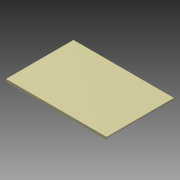
# Autodesk Inventor part: SidePanelNarrow
Saved by Autodesk Inventor 2015 (Build 190159000, 159)
## iProperties
Created: 2015-04-21
Part Number: SidePanelNarrow
Material: Nylon 6
Document SubType Name: Modeling
Designer: Akovo_000
Mass: 17.0375 g
Surface Area: 300.154 cm^2
Volume: 15.2121 cm^3
Density: 1.12 g/cm^3
Appearance: Nylon 6
Author: Akovo_000
Autodesk Inventor part; units mm, degrees
ref_plane "YZ Plane" through (0, 0, 0) normal (1, 0, 0) x (0, 1, 0)
ref_plane "XZ Plane" through (0, 0, 0) normal (0, 1, 0) x (-1, 0, 0)
ref_plane "XY Plane" through (0, 0, 0) normal (0, 0, 1) x (1, 0, 0)
sketch "PanelBody" plane through (0, 0, 0) normal (0, 0, 1) x (1, 0, 0)
  line L0 (-106.0995, -38.4223) -> (33.9005, -38.4223)
  line L1 (33.9005, -38.4223) -> (33.9005, -132.4223)
  line L2 (33.9005, -132.4223) -> (-106.0995, -132.4223)
  line L3 (-106.0995, -132.4223) -> (-106.0995, -38.4223)
  dimension "d1" = 140
  dimension "d2" = 94
  constraints: 8 end point, 2 parallel, 1 horizontal, 1 perpendicular
  measures "d1" distance of L1.end L2.end
  measures "d2" distance of L0.end L1.end
extrude "PanelFace" add sketch "PanelBody" along normal blind 2
sketch "SideHooks" plane through (-106.0995, -132.4223, 0) normal (-1, 0, 0) x (0, 0, 1)
  line L0 (0, 94) -> (-1.9, 94)
  line L1 (-1.9, 94) -> (-1.9, 92.1)
  line L2 (-1.9, 92.1) -> (0, 92.1)
  line L3 (0, 92.1) -> (0, 94)
  line L4 (0, 0) -> (-1.9, 0)
  line L5 (-1.9, 0) -> (-1.9, 1.9)
  line L6 (-1.9, 1.9) -> (0, 1.9)
  line L7 (0, 1.9) -> (0, 0)
  point P0 (0, 132.4223)
  dimension "d33" = 1.9
  constraints: 16 end point, 4 parallel, 3 equal length, 2 horizontal, 2 perpendicular
  measures "d33" distance of L5.end L6.end
extrude "Corners" add sketch "SideHooks" against normal blind 140
sketch "Sketch3" plane through (33.9005, -38.4223, -1.9) normal (0, 0, -1) x (-1, 0, 0)
  line L0 (0, -94) -> (140, -94) construction
  line L1 (140, -94) -> (140, 0) construction
  line L2 (140, 0) -> (0, 0) construction
  line L3 (0, 0) -> (0, -94) construction
  line L4 (137.5, -91.5) -> (133.8633, -91.5) construction
  line L5 (72.5, -86.5) -> (72.5, -56.6362)
  line L6 (137.5, -54.5) -> (137.5, -85.1873)
  line L7 (137.5, -2.5) -> (133.8633, -2.5) construction
  line L8 (72.5, -7.5) -> (72.5, -37.3638)
  line L9 (137.5, -39.5) -> (137.5, -8.8127)
  line L10 (2.5, -2.5) -> (6.1367, -2.5) construction
  line L11 (67.5, -7.5) -> (67.5, -37.3638)
  line L12 (2.5, -39.5) -> (2.5, -8.8127)
  line L13 (2.5, -91.5) -> (6.1367, -91.5) construction
  line L14 (67.5, -86.5) -> (67.5, -56.6362)
  line L15 (2.5, -54.5) -> (2.5, -85.1873)
  line L16 (72.5, -2.5) -> (67.5, -2.5) construction
  line L17 (2.5, -44.5) -> (2.5, -49.5) construction
  line L18 (67.5, -91.5) -> (72.5, -91.5) construction
  line L19 (137.5, -44.5) -> (137.5, -49.5) construction
  line L20 (135.2172, -7.5332) -> (79.3341, -41.7204)
  line L21 (74.7828, -38.6434) -> (129.3198, -5.2796)
  line L22 (65.2172, -38.6434) -> (10.6802, -5.2796)
  line L23 (60.6659, -41.7204) -> (4.7828, -7.5332)
  line L24 (11.4629, -2.5) -> (62.5, -2.5)
  line L25 (2.5, -6.1367) -> (2.5, -2.5) construction
  line L26 (80.1169, -44.5) -> (132.5, -44.5)
  line L27 (137.5, -6.1367) -> (137.5, -2.5) construction
  line L28 (128.5371, -2.5) -> (77.5, -2.5)
  line L29 (59.8831, -44.5) -> (7.5, -44.5)
  line L30 (135.2172, -86.4668) -> (79.3341, -52.2796)
  line L31 (74.7828, -55.3566) -> (129.3198, -88.7204)
  line L32 (65.2172, -55.3566) -> (10.6802, -88.7204)
  line L33 (4.7828, -86.4668) -> (60.6659, -52.2796)
  line L34 (80.1169, -49.5) -> (132.5, -49.5)
  line L35 (59.8831, -49.5) -> (7.5, -49.5)
  line L36 (2.5, -87.8633) -> (2.5, -91.5) construction
  line L37 (11.4629, -91.5) -> (62.5, -91.5)
  line L38 (128.5371, -91.5) -> (77.5, -91.5)
  line L39 (137.5, -87.8633) -> (137.5, -91.5) construction
  line L40 (140, -94) -> (0, -94) projected
  line L41 (140, 0) -> (0, 0) projected
  line L42 (0, -1.9) -> (0, -92.1) projected
  line L43 (140, 0) -> (140, -1.9) projected
  line L44 (103.0028, -27.2408) -> (100.3935, -22.9756) construction
  line L45 (91.7427, -59.8707) -> (89.1334, -64.1358) construction
  line L46 (57.5593, -60.0415) -> (54.95, -55.7763) construction
  line L47 (48.3721, -34.1995) -> (50.9813, -29.9344) construction
  line L48 (74.7906, -49.5) -> (65.2094, -49.5) construction
  line L49 (65.2094, -44.5) -> (74.7906, -44.5) construction
  line L50 (72.5, -53.9601) -> (72.5, -40.0399) construction
  line L51 (67.5, -53.9601) -> (67.5, -40.0399) construction
  arc A0 (77.5, -2.5) -> (72.5, -7.5) centre (77.5, -7.5) ccw
  arc A1 (67.5, -7.5) -> (62.5, -2.5) centre (62.5, -7.5) ccw
  arc A2 (72.5, -86.5) -> (77.5, -91.5) centre (77.5, -86.5) ccw
  arc A3 (62.5, -91.5) -> (67.5, -86.5) centre (62.5, -86.5) ccw
  arc A4 (2.5, -39.5) -> (7.5, -44.5) centre (7.5, -39.5) ccw
  arc A5 (7.5, -49.5) -> (2.5, -54.5) centre (7.5, -54.5) ccw
  arc A6 (137.5, -54.5) -> (132.5, -49.5) centre (132.5, -54.5) ccw
  arc A7 (132.5, -44.5) -> (137.5, -39.5) centre (132.5, -39.5) ccw
  arc A8 (80.1169, -49.5) -> (79.3341, -52.2796) centre (80.1169, -51) ccw
  arc A9 (74.7828, -55.3566) -> (72.5, -56.6362) centre (74, -56.6362) ccw
  arc A10 (67.5, -56.6362) -> (65.2172, -55.3566) centre (66, -56.6362) ccw
  arc A11 (60.6659, -52.2796) -> (59.8831, -49.5) centre (59.8831, -51) ccw
  arc A12 (59.8831, -44.5) -> (60.6659, -41.7204) centre (59.8831, -43) ccw
  arc A13 (65.2172, -38.6434) -> (67.5, -37.3638) centre (66, -37.3638) ccw
  arc A14 (72.5, -37.3638) -> (74.7828, -38.6434) centre (74, -37.3638) ccw
  arc A15 (79.3341, -41.7204) -> (80.1169, -44.5) centre (80.1169, -43) ccw
  arc A16 (137.5, -8.8127) -> (135.2172, -7.5332) centre (136, -8.8127) ccw
  arc A17 (129.3198, -5.2796) -> (128.5371, -2.5) centre (128.5371, -4) ccw
  arc A18 (11.4629, -2.5) -> (10.6802, -5.2796) centre (11.4629, -4) ccw
  arc A19 (4.7828, -7.5332) -> (2.5, -8.8127) centre (4, -8.8127) ccw
  arc A20 (2.5, -85.1873) -> (4.7828, -86.4668) centre (4, -85.1873) ccw
  arc A21 (10.6802, -88.7204) -> (11.4629, -91.5) centre (11.4629, -90) ccw
  arc A22 (128.5371, -91.5) -> (129.3198, -88.7204) centre (128.5371, -90) ccw
  arc A23 (135.2172, -86.4668) -> (137.5, -85.1873) centre (136, -85.1873) ccw
  dimension "d16" = 2.5
  dimension "d24" = 5
  dimension "d25" = 5
  dimension "d26" = 2.5
  dimension "d27" = 2.5
  dimension "d28" = 2.5
  dimension "d34" = 0
  dimension "d36" = 0
  dimension "d37" = 0
  dimension "d38" = 0
  dimension "d39" = 5
  dimension "d40" = 5
  dimension "d41" = 1.5
  constraints: 96 end point, 57 point on line, 48 point on circle, 48 tangent, 24 centre point, 22 equal radius, 14 equal length, 12 horizontal, 12 vertical, 6 collinear, 6 parallel, 6 perpendicular
  measures "d16" distance between parallel lines of L10 L2
  measures "d24" distance between parallel lines of L20 L21
  measures "d25" distance of L17.start L17.end
  measures "d26" horizontal distance of L0.start L13.start
  measures "d27" horizontal distance of L1.end L7.start
  measures "d28" horizontal distance of L0.end L4.start
  measures "d34" distance from line of L40 L0.start
  measures "d36" distance between parallel lines of L41 L2
  measures "d37" distance between parallel lines of L42 L3
  measures "d38" distance between parallel lines of L43 L1
  measures "d39" distance between parallel lines of L5 L14
  measures "d40" radius of A0
  measures "d41" radius of A8
extrude "ReinforcementBars" cut sketch "Sketch3" against normal blind 3.2
sketch "Sketch4" plane through (0, 0, 2) normal (0, 0, 1) x (1, 0, 0)
  line L0 (-62.4757, -113.2868) -> (-62.4757, -58.6034) construction
  line L1 (-62.4757, -58.6034) -> (1.9126, -58.6034) construction
  line L2 (1.9126, -58.6034) -> (1.9126, -113.2868) construction
  line L3 (1.9126, -113.2868) -> (-62.4757, -113.2868) construction
  point P0 (0, 0)
  constraints: 2 other
extrude "Extrusion4" [suppressed]
body "Solid1"
